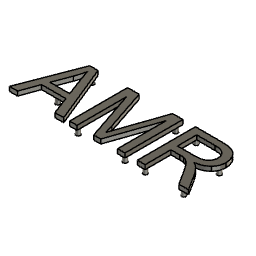
AMR로고 (Autodesk Fusion 360 design; units mm, degrees)
Autodesk Fusion 360 part; units mm, degrees
note: some values were not read from the file. Set by a fixed rule: which sketch regions a step uses.
sketch "스케치1" plane through (0, 0, 0) normal (0, 0, 1) x (1, 0, 0)
  line L0 (-55.25, 87.25) -> (-55.25, 72.75)
  line L1 (-55.25, 72.75) -> (-28.25, 72.75)
  line L2 (-28.25, 72.75) -> (-28.25, 87.25)
  line L3 (-28.25, 87.25) -> (-55.25, 87.25)
  line L4 (-28.25, 72.75) -> (-2.75, 72.75)
  line L5 (-28.25, 72.75) -> (-28.25, 49.25)
  line L6 (-2.75, 72.75) -> (29.75, 72.75)
  line L7 (-2.75, 72.75) -> (-2.75, 37.75)
  line L8 (43.75, 72.75) -> (43.75, 37.75)
  line L9 (29.75, 72.75) -> (29.75, 37.75)
  line L10 (69.75, 72.75) -> (43.75, 72.75)
  line L11 (69.75, 62.75) -> (69.75, 72.75)
  line L12 (43.75, 37.75) -> (70.25, 37.75)
  line L13 (-55.25, 87.25) -> (84.75, 87.25)
  line L14 (84.75, 22.25) -> (-55.25, 22.25)
  line L15 (-55.25, 22.25) -> (-55.25, 87.25)
  line L16 (84.75, 87.25) -> (84.75, 22.25)
  circle A0 centre (-28.25, 72.75) radius 1.5
  circle A1 centre (-28.25, 49.25) radius 1.5
  circle A2 centre (-2.75, 72.75) radius 1.5
  circle A3 centre (-2.75, 37.75) radius 1.5
  circle A4 centre (29.75, 72.75) radius 1.5
  circle A5 centre (29.75, 37.75) radius 1.5
  circle A6 centre (69.75, 62.75) radius 1.5
  circle A7 centre (43.75, 72.75) radius 1.5
  circle A8 centre (43.75, 37.75) radius 1.5
  circle A9 centre (70.25, 37.75) radius 1.5
  line L17 (-55.25, 22.25) -> (84.75, 22.25) construction
  line L18 (84.75, 22.25) -> (84.75, 87.25) construction
  line L19 (84.75, 87.25) -> (-55.25, 87.25) construction
  line L20 (-55.25, 87.25) -> (-55.25, 22.25) construction
  dimension "d3" = 65
  dimension "d4" = 140
  dimension "d5" = 23.5
  dimension "d6" = 25.5
  dimension "d7" = 26.5
  dimension "d8" = 3
  dimension "d9" = 3
  dimension "d10" = 3
  dimension "d11" = 3
  dimension "d12" = 3
  dimension "d13" = 3
  dimension "d14" = 3
  dimension "d15" = 3
  dimension "d16" = 3
  dimension "d17" = 3
  dimension "d20" = 40
  text T0 "AMR" font "Arial" height 40 align centre middle in box 140 x 65 at (-55.25, 22.25) x (1, 0) y (0, 1) spacing 1
  constraint perpendicular L14 L16
  constraint parallel L15 L16
  constraint parallel L13 L14
  constraint perpendicular L1 L5
  constraint parallel L1 L4
  constraint perpendicular L6 L7
  constraint perpendicular L6 L9
  constraint parallel L8 L9
  constraint perpendicular L8 L12
  constraint coincident L1.end L2.start
  constraint coincident L5.end A1.centre
  constraint coincident L4.end L6.start
  constraint coincident L7.end A3.centre
  constraint coincident L6.end L9.start
  constraint coincident L9.end A5.centre
  constraint coincident L11.start A6.centre
  constraint coincident L8.start L10.end
  constraint coincident L8.end L12.start
  constraint coincident L12.end A9.centre
  constraint coincident L14.start
  constraint coincident L0.start
  measures "d3" distance of L0.start L14.end
  measures "d4" distance of L14.start L14.end
  measures "d5" distance of L5.end L1.end
  measures "d6" distance of L1.end L4.end
  measures "d7" distance of L8.end L12.end
  measures "d8" diameter of A0
  measures "d9" diameter of A1
  measures "d10" diameter of A2
  measures "d11" diameter of A3
  measures "d12" diameter of A4
  measures "d13" diameter of A5
  measures "d14" diameter of A6
  measures "d15" diameter of A7
  measures "d16" diameter of A8
  measures "d17" diameter of A9
extrude "돌출1" add sketch "스케치1" against normal blind 5 contours L1 L2 A0 | L1 L5 A0 | L2 L4 A0 | L4 L5 A0 | L4 L6 A2 | L4 L7 A2 | L6 L7 A2 | L6 L9 A4 | L6 L9 A4 | L8 L10 A7 | L8 L10 A7 | L8 L12 A8 | L8 L12 A8 | A1 | A3 | A5 | A6 | A9 makes body 1 at (45.1322, 38.3327, -1.6667) makes body 2 at (-1.3678, 38.3327, -1.6667) makes body 3 at (-29.6595, 73.263, -3.3333) makes body 4 at (31.2036, 38.1201, -1.6667) makes body 5 at (71.6322, 38.3327, -1.6667) makes body 6 at (45.1595, 72.237, -1.6667) makes body 7 at (-1.3405, 72.237, -1.6667) makes body 8 at (-26.8678, 49.8327, -1.6667) makes body 9 at (31.1595, 73.263, -3.3333) makes body 10 at (69.4895, 61.2728, -1.6667)
extrude "돌출2" add sketch "스케치1" along normal blind 3 text T0 bodies 1 2 3 4 5 6 7 8 9 10
